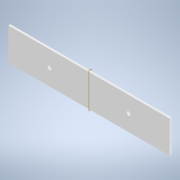
# Autodesk Inventor part: Wheel Posts Mount
Saved by Autodesk Inventor 2022 (Build 260153000, 153)
## iProperties
Created: 2022-01-21
Part Number: Wheel Posts Mount
Material: Generic
Document SubType Name: Modeling
Designer: gnzak
Density: 1 g/cm^3
Appearance: Default
Author: gnzak
Autodesk Inventor part; units mm, degrees
ref_plane "YZ Plane" through (0, 0, 0) normal (1, 0, 0) x (0, 1, 0)
ref_plane "XZ Plane" through (0, 0, 0) normal (0, 1, 0) x (-1, 0, 0)
ref_plane "XY Plane" through (0, 0, 0) normal (0, 0, 1) x (1, 0, 0)
sketch "Sketch1" plane through (0, 0, 0) normal (0, 0, 1) x (1, 0, 0)
  line L0 (-55.8352, 26.7427) -> (198.1648, 26.7427)
  line L1 (198.1648, 26.7427) -> (198.1648, -24.0573)
  line L2 (198.1648, -24.0573) -> (-55.8352, -24.0573)
  line L3 (-55.8352, -24.0573) -> (-55.8352, 26.7427)
  circle A0 centre (8.9348, 1.3427) radius 3.175
  circle A1 centre (133.3948, 1.3427) radius 3.175
  point P0 (0, 0)
  dimension "d0" = 50.8
  dimension "d1" = 254
  dimension "d2" = 124.46
  dimension "d3" = 6.35
  dimension "d4" = 6.35
  dimension "d5" = 25.4
  dimension "d6" = 25.4
  dimension "d8" = 64.77
  constraints: 8 end point, 2 centre point, 2 parallel, 1 horizontal, 1 perpendicular
  measures "d0" distance of L2.end L0.start
  measures "d1" distance of L0.start L0.end
  measures "d2" distance of A1.centre A0.centre
  measures "d3" diameter of A1
  measures "d4" diameter of A0
  measures "d5" distance from line of L0 A0.centre
  measures "d6" distance from line of L0 A1.centre
  measures "d8" distance from line of L3 A0.centre
extrude "Extrusion1" add sketch "Sketch1" along normal blind 3.175
ref_plane "Work Plane1" through (71.1648, -24.0573, 0) normal (1, 0, 0) x (0, 0, -1)
equation "\"d5\" = 0.5 * d0"
equation "\"d6\" = 0.5 * d0"
equation "\"d8\" = -0.5 * d2 + 0.5 * d1"
body "Solid1"
